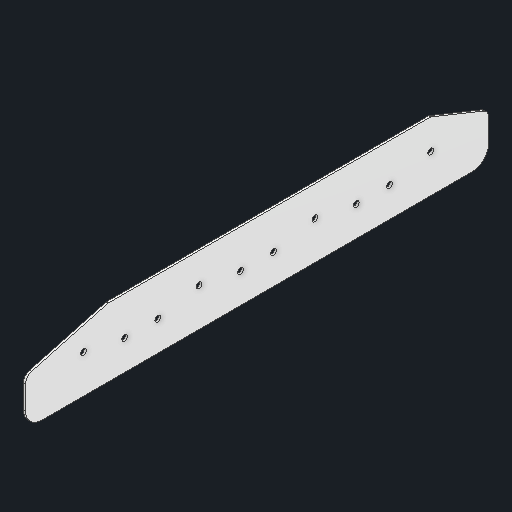
# Autodesk Inventor part: Skirt
Saved by Autodesk Inventor 2025 (Build 290162000, 162)
## iProperties
Created: 2024-12-17
Part Number: Skirt
Material: Acetal Resin, White
Document SubType Name: Modeling
Designer: Averey Ku
Density: 1.425 g/cm^3
Appearance: Smooth - White
Author: Averey Ku
Autodesk Inventor part; units mm, degrees
ref_plane "YZ Plane" through (0, 0, 0) normal (1, 0, 0) x (0, 1, 0)
ref_plane "XZ Plane" through (0, 0, 0) normal (0, 1, 0) x (-1, 0, 0)
ref_plane "XY Plane" through (0, 0, 0) normal (0, 0, 1) x (1, 0, 0)
sketch "main" plane through (0, 0, 0) normal (0, 0, 1) x (1, 0, 0)
  circle A0 centre (5.8723, 139.0371) radius 2.1844
  arc A1 (-10.7964, 183.4871) -> (-23.4964, 170.7871) centre (-10.7964, 170.7871) ccw
  circle A2 centre (-0.4777, 107.2871) radius 2.1844
  line L0 (12.9013, 178.803) -> (28.8911, 119.9871)
  line L1 (-10.7964, 183.4871) -> (6.7737, 183.4871)
  arc A3 (12.9013, 178.803) -> (6.7737, 183.4871) centre (6.7737, 177.1371) ccw
  circle A4 centre (5.8723, 50.1371) radius 2.1844
  circle A5 centre (5.8723, -38.7629) radius 2.1844
  circle A6 centre (5.8723, -127.6629) radius 2.1844
  circle A7 centre (-0.4777, 81.8871) radius 2.1844
  circle A8 centre (-0.4777, 18.3871) radius 2.1844
  line L2 (-23.4964, -159.4129) -> (-23.4964, 170.7871)
  line L3 (28.8911, 119.9871) -> (28.8911, -127.6629)
  circle A9 centre (-0.4777, -70.5129) radius 2.1844
  circle A10 centre (-0.4777, -95.9129) radius 2.1844
  line L4 (12.5958, -168.1346) -> (28.8911, -127.6629)
  arc A11 (6.7053, -172.1129) -> (12.5958, -168.1346) centre (6.7053, -165.7629) ccw
  line L5 (6.7053, -172.1129) -> (9.8411, -172.1129)
  line L6 (-10.7964, -172.1129) -> (6.7053, -172.1129)
  arc A12 (-23.4964, -159.4129) -> (-10.7964, -172.1129) centre (-10.7964, -159.4129) ccw
  circle A13 centre (-0.4777, -7.0129) radius 2.1844
  point P0 (2.0753, 1.669)
  dimension "d0" = 6.35
  dimension "d1" = 6.35
  measures "d0" radius of A3
  measures "d1" radius of A11
sketch "Sketch1" plane through (0, 0, 0) normal (1, 0, 0) x (0, 1, 0)
  circle A0 centre (0, 0) radius 2.1844
  arc A1 (-16.6688, 44.45) -> (-29.3688, 31.75) centre (-16.6688, 31.75) ccw
  circle A2 centre (-6.35, -31.75) radius 2.1844
  line L0 (7.029, 39.7659) -> (23.0187, -19.05)
  line L1 (-16.6688, 44.45) -> (0.9014, 44.45)
  arc A3 (7.029, 39.7659) -> (0.9014, 44.45) centre (0.9014, 38.1) ccw
  circle A4 centre (0, -88.9) radius 2.1844
  circle A5 centre (0, -177.8) radius 2.1844
  circle A6 centre (0, -266.7) radius 2.1844
  circle A7 centre (-6.35, -57.15) radius 2.1844
  circle A8 centre (-6.35, -120.65) radius 2.1844
  line L2 (-29.3688, -298.45) -> (-29.3688, 31.75)
  line L3 (23.0187, -19.05) -> (23.0187, -266.7)
  circle A9 centre (-6.35, -209.55) radius 2.1844
  circle A10 centre (-6.35, -234.95) radius 2.1844
  line L4 (6.7235, -307.1717) -> (23.0187, -266.7)
  arc A11 (0.833, -311.15) -> (6.7235, -307.1717) centre (0.833, -304.8) ccw
  line L5 (0.833, -311.15) -> (3.9687, -311.15)
  line L6 (-16.6688, -311.15) -> (0.833, -311.15)
  arc A12 (-29.3688, -298.45) -> (-16.6688, -311.15) centre (-16.6688, -298.45) ccw
  circle A13 centre (-6.35, -146.05) radius 2.1844
  constraints: 1 other
extrude "Extrusion1" add sketch "Sketch1" along normal blind 1.5875
body "Solid1"
